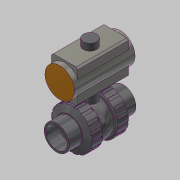
# Autodesk Inventor part: BALL VALVE PNEUMATIC GLUED DN50
Saved by Autodesk Inventor 2017 (Build 210142000, 142)
## iProperties
Created: 2016-04-26
Part Number: BALL VALVE PNEUMATIC GLUED DN50
Description: DUAL BLOCK VINK
Document SubType Name: Modeling
Manufacturer: SEKISUI
Mass: 197.859 g
Surface Area: 285.44 cm^2
Volume: 153.379 cm^3
Density: 1.29 g/cm^3
Material: U-PVC
Appearance: Smooth - Medium Gray
Title: BALL VALVE PVC-U TRD DN15
Autodesk Inventor part; units mm, degrees
ref_plane "YZ Plane" through (0, 0, 0) normal (1, 0, 0) x (0, 1, 0)
ref_plane "XZ Plane" through (0, 0, 0) normal (0, 1, 0) x (-1, 0, 0)
ref_plane "XY Plane" through (0, 0, 0) normal (0, 0, 1) x (1, 0, 0)
sketch "Sketch_1" plane through (0, 0, 0) normal (0, 0, 1) x (1, 0, 0)
  line L0 (61.5, 0) -> (61.5, -40.6667)
  line L1 (61.5, -40.6667) -> (54.0993, -61)
  line L2 (54.0993, -61) -> (22.4048, -61)
  line L3 (22.4048, -61) -> (20.5, -55.7667)
  line L4 (20.5, -55.7667) -> (20.5, -50.1976)
  arc A0 (-20.5, -50.1976) -> (20.5, -50.1976) centre (0, 0) ccw
  line L5 (-20.5, -50.1976) -> (-20.5, -55.7667)
  line L6 (-20.5, -55.7667) -> (-22.4048, -61)
  line L7 (-22.4048, -61) -> (-54.0993, -61)
  line L8 (-54.0993, -61) -> (-61.5, -40.6667)
  line L9 (-61.5, -40.6667) -> (-61.5, 0)
  line L10 (-61.5, 0) -> (61.5, 0)
  line L11 (-22.4048, -61) -> (0, -61) construction
  line L12 (0, -61) -> (0, -54.2222) construction
  line L13 (-54.8272, -61) -> (-24.4048, -61)
  line L14 (-24.4048, -61) -> (-24.4048, -59)
  line L15 (-24.4048, -59) -> (-54.8272, -59)
  line L16 (-54.8272, -59) -> (-54.8272, -61)
  line L17 (24.4048, -61) -> (54.8272, -61)
  line L18 (54.8272, -61) -> (54.8272, -59)
  line L19 (54.8272, -59) -> (24.4048, -59)
  line L20 (24.4048, -59) -> (24.4048, -61)
  point P0 (-38.252, -61)
  dimension "dimZ" = 123
  dimension "dimE" = 122
  dimension "d22" = 61
  dimension "d23" = 20.3333
  dimension "d24" = 20
  dimension "d27" = 41
  dimension "d28" = 41
  dimension "d40" = 6.7778
  dimension "d52" = 20
  dimension "d53" = 2
  dimension "d54" = 2
  dimension "d55" = 2
  constraints: 42 end point, 6 parallel, 5 equal length, 5 perpendicular, 4 horizontal, 3 collinear, 3 point on circle, 3 point on line, 2 coincident, 2 midpoint, 1 centre point
  measures "dimZ" distance of L9.end L0.start
  measures "dimE" diameter of L2 L10
  measures "d22" distance from line of L0.start L2
  measures "d23" vertical distance of L0.end L1.end
  measures "d24" angle of L0 L1
  measures "d27" distance between parallel lines of L9 L5
  measures "d28" distance between parallel lines of L0 L4
  measures "d40" distance of L11.end L12.end
  measures "d52" angle of L5 L6
  measures "d53" distance of L15.end L13.start
  measures "d54" distance from line of L6.end L14
  measures "d55" distance from line of L2.end L20
revolve "Revolution1" add sketch "Sketch_1" angle 360 about axis through (-61.5, 0, 0) along (1, 0, 0) contours L0 L1 L19 L20 L2 L3 L4 A0 L5 L6 L7 L14 L15 L8 L9 L10 | L1 L2 L20 L19 | L15 L14 L7 L8
sketch "Sketch_2" plane through (0, 0, 0) normal (0, 0, 1) x (1, 0, 0)
  line L0 (0, 0) -> (0, 88)
  line L1 (0, 88) -> (20.5, 88)
  line L2 (20.5, 88) -> (20.5, 0)
  line L3 (20.5, 0) -> (0, 0)
  line L4 (0, 0) -> (0, 88)
  line L5 (20.5, -55.7667) -> (20.5, 55.7667) projected
  dimension "dimB" = 88
  constraints: 10 end point, 2 perpendicular, 1 coincident, 1 collinear, 1 vertical
  measures "dimB" distance of L0.start L0.end
revolve "Revolution2" add sketch "Sketch_2" angle 360 about axis through (0, 0, 0) along (0, -1, 0)
sketch "Sketch_7" plane through (0, 0, 0) normal (0, 0, 1) x (1, 0, 0)
  line L0 (-99.5, 37.5) -> (99.5, 37.5)
  line L1 (48.5126, 0) -> (-48.5126, 0)
  line L2 (-99.5, 37.5) -> (-99.5, 31.5)
  line L3 (-99.5, 31.5) -> (99.5, 31.5)
  line L4 (99.5, 31.5) -> (99.5, 37.5)
  line L5 (0, -7.5) -> (0, 45) projected
  point P0 (0, 0)
  point P1 (0, 0)
  point P2 (0, 31.5)
  dimension "dimH" = 199
  dimension "dimD" = 63
  dimension "dimD2" = 75
  constraints: 10 end point, 2 midpoint, 2 perpendicular, 1 coincident, 1 horizontal, 1 parallel, 1 point on line, 1 vertical
  measures "dimH" distance of L2.end L3.end
  measures "dimD" diameter of L3 L1
  measures "dimD2" diameter of L0 L1
revolve "Revolution3" add sketch "Sketch_7" angle 360 about axis through (48.5126, 0, 0) along (-1, 0, 0)
extrude "Extrusion8" cut sketch "Sketch_1" along normal mid plane 8.1333 contours L18 L17 L1 | L1 L2 L20 L19 | L15 L14 L7 L8 | L8 L13 L16
pattern_circular "Circular Pattern1" count 17 over 360 about axis through (49.75, 0, 0) along (-1, 0, 0) of "Extrusion8"
sketch "Sketch15" plane through (0, 0, 0) normal (1, 0, 0) x (0, 1, 0)
  line L0 (88, -39) -> (88, 39)
  line L1 (88, 39) -> (188, 39)
  line L2 (188, 39) -> (188, -39)
  line L3 (188, -39) -> (88, -39)
  line L4 (188, 39) -> (88, -39) construction
  line L5 (188, -39) -> (88, 39) construction
  circle A0 centre (138, 0) radius 44
  line L6 (188, 0) -> (188, 20)
  line L7 (188, 20) -> (208, 20)
  line L8 (208, 20) -> (208, 0)
  line L9 (208, 0) -> (188, 0)
  circle A1 centre (0, 0) radius 37.5 projected
  line L10 (0, 0) -> (138, 0)
  line L11 (88, 20.5) -> (88, -20.5) projected
  point P0 (0, 0)
  dimension "oActuatorWidth" = 78
  dimension "oActuatorHeight" = 100
  dimension "oActuatorDiam" = 88
  dimension "d62" = 20
  dimension "d63" = 20
  constraints: 22 end point, 4 parallel, 3 midpoint, 3 perpendicular, 2 vertical, 1 centre point, 1 collinear
  measures "oActuatorWidth" distance of L1.end L2.end
  measures "oActuatorHeight" distance of L0.end L1.end
  measures "oActuatorDiam" diameter of A0
  measures "d62" distance of L7.end L8.end
  measures "d63" distance of L6.end L7.end
extrude "Extrusion9" add sketch "Sketch15" along normal mid plane 181 contours A0 L1 L3 | L3 A0 | A0 L1
extrude "Extrusion10" add sketch "Sketch15" along normal mid plane 151 contours L0 L10 A0 L3 | A0 L1 L3 | L0 L1 A0 L10 | A0 L1 L2 L3
revolve "Revolution6" add sketch "Sketch15" angle 360 about axis through (0, 208, 0) along (0, -1, 0) contours L2 L7 L8 L9
chamfer "Chamfer1" distance 5 angle 45 4 edges at (0, 188, -39) (0, 188, 39) (0, 88, 39) (0, 88, -39)
equation "\"d23\" = 0.333333 * d22"
equation "\"d27\" = 0.333333 * dimZ"
equation "\"d28\" = d27"
equation "\"d40\" = 0.333333 * d23"
equation "\"d47\" = 0.0666667 * dimE"
equation "\"oMe\" = dimE"
body "Solid1"
